Autodesk Fusion 360 part; units mm, degrees
note: some values were not read from the file. Set by a fixed rule: which face or edge a step refers to.
(part 5 of 12)
sketch "Sketch1" plane through (0, 0, 0) normal (0, 0, 1) x (1, 0, 0) in component "Component"
  spline S0 degree 5 poles (6.0486, -1.3928) (6.0487, -1.3928) (6.049, -1.3929) (6.0495, -1.393) (6.0503, -1.3931) (6.0514, -1.3934) (6.0527, -1.3936) (6.0541, -1.3939) (6.0558, -1.3942) (6.0576, -1.3945) (6.0596, -1.3948) (6.0618, -1.3952) (6.0641, -1.3955) (6.0665, -1.3959) (6.0692, -1.3963) (6.072, -1.3967) (6.0749, -1.3971) (6.078, -1.3975) (6.0812, -1.3979) (6.0846, -1.3983) (6.0881, -1.3987) (6.0918, -1.3991) (6.0956, -1.3995) (6.0995, -1.3999) (6.1036, -1.4002) (6.1078, -1.4006) (6.1121, -1.401) (6.1166, -1.4013) (6.1212, -1.4017) (6.1259, -1.402) (6.1308, -1.4023) (6.1357, -1.4026) (6.1408, -1.4029) (6.1461, -1.4032) (6.1514, -1.4034) (6.1569, -1.4036) (6.1624, -1.4038) (6.1681, -1.404) (6.1739, -1.4041) (6.1798, -1.4043) (6.1858, -1.4044) (6.192, -1.4044) (6.1982, -1.4045) (6.2046, -1.4045) (6.211, -1.4045) (6.2176, -1.4045) (6.2242, -1.4044) (6.231, -1.4043) (6.2379, -1.4042) (6.2448, -1.404) (6.2519, -1.4038) (6.259, -1.4036) (6.2663, -1.4033) (6.2736, -1.403) (6.2811, -1.4026) (6.2886, -1.4022) (6.2962, -1.4018) (6.304, -1.4014) (6.3118, -1.4009) (6.3197, -1.4003) (6.3277, -1.3997) (6.3357, -1.3991) (6.3439, -1.3985) (6.3522, -1.3978) (6.3605, -1.397) (6.3689, -1.3962) (6.3774, -1.3954) (6.386, -1.3945) (6.3946, -1.3936) (6.4034, -1.3926) (6.4122, -1.3916) (6.4211, -1.3905) (6.43, -1.3894) (6.4391, -1.3882) (6.4482, -1.387) (6.4574, -1.3858) (6.4667, -1.3845) (6.476, -1.3831) (6.4855, -1.3817) (6.4949, -1.3803) (6.5045, -1.3788) (6.5141, -1.3772) (6.5238, -1.3756) (6.5336, -1.3739) (6.5434, -1.3722) (6.5533, -1.3704) (6.5633, -1.3686) (6.5733, -1.3668) (6.5834, -1.3648) (6.5936, -1.3628) (6.6038, -1.3608) (6.6141, -1.3587) (6.6244, -1.3566) (6.6348, -1.3544) (6.6453, -1.3521) (6.6558, -1.3498) (6.6664, -1.3474) (6.6771, -1.345) (6.6878, -1.3425) (6.6985, -1.34) (6.7093, -1.3374) (6.7202, -1.3347) (6.7311, -1.332) (6.7421, -1.3292) (6.7531, -1.3264) (6.7642, -1.3235) (6.7754, -1.3206) (6.7865, -1.3176) (6.7978, -1.3145) (6.8091, -1.3114) (6.8204, -1.3082) (6.8318, -1.3049) (6.8432, -1.3016) (6.8547, -1.2982) (6.8663, -1.2948) (6.8778, -1.2913) (6.8895, -1.2878) (6.9011, -1.2842) (6.9129, -1.2805) (6.9246, -1.2767) (6.9364, -1.2729) (6.9483, -1.2691) (6.9602, -1.2651) (6.9721, -1.2611) (6.9841, -1.2571) (6.9961, -1.253) (7.0081, -1.2488) (7.0202, -1.2445) (7.0324, -1.2402) (7.0445, -1.2359) (7.0568, -1.2314) (7.069, -1.2269) (7.0813, -1.2224) (7.0936, -1.2177) (7.106, -1.213) (7.1184, -1.2083) (7.1308, -1.2035) (7.1433, -1.1986) (7.1558, -1.1936) (7.1683, -1.1886) (7.1809, -1.1835) (7.1935, -1.1784) (7.2061, -1.1731) (7.2188, -1.1679) (7.2314, -1.1625) (7.2442, -1.1571) (7.2569, -1.1516) (7.2697, -1.1461) (7.2825, -1.1405) (7.2953, -1.1348) (7.3082, -1.129) (7.3211, -1.1232) (7.334, -1.1173) (7.347, -1.1114) (7.36, -1.1054) (7.373, -1.0993) (7.386, -1.0932) (7.399, -1.0869) (7.4121, -1.0807) (7.4252, -1.0743) (7.4383, -1.0679) (7.4515, -1.0614) (7.4646, -1.0549) (7.4778, -1.0482) (7.491, -1.0416) (7.5043, -1.0348) (7.5175, -1.028) (7.5308, -1.0211) (7.5441, -1.0141) (7.5574, -1.0071) (7.5707, -1) (7.5841, -0.9929) (7.5974, -0.9856) (7.6108, -0.9783) (7.6242, -0.971) (7.6376, -0.9635) (7.6511, -0.956) (7.6645, -0.9484) (7.678, -0.9408) (7.6914, -0.9331) (7.7049, -0.9253) (7.7184, -0.9175) (7.732, -0.9096) (7.7455, -0.9016) (7.759, -0.8935) (7.7726, -0.8854) (7.7862, -0.8772) (7.7998, -0.869) (7.8134, -0.8606) (7.827, -0.8523) (7.8406, -0.8438) (7.8542, -0.8353) (7.8678, -0.8267) (7.8815, -0.818) (7.8951, -0.8093) (7.9088, -0.8004) (7.9225, -0.7916) (7.9361, -0.7826) (7.9498, -0.7736) (7.9635, -0.7645) (7.9772, -0.7554) (7.9909, -0.7462) (8.0046, -0.7369) (8.0183, -0.7275) (8.0321, -0.7181) (8.0458, -0.7086) (8.0595, -0.6991) (8.0732, -0.6894) (8.087, -0.6797) (8.1007, -0.67) (8.1145, -0.6601) (8.1282, -0.6502) (8.1419, -0.6402) (8.1557, -0.6302) (8.1694, -0.6201) (8.1832, -0.6099) (8.1969, -0.5997) (8.2107, -0.5894) (8.2244, -0.579) (8.2382, -0.5685) (8.2519, -0.558) (8.2657, -0.5474) (8.2794, -0.5368) (8.2932, -0.526) (8.3069, -0.5152) (8.3207, -0.5044) (8.3344, -0.4934) (8.3481, -0.4824) (8.3619, -0.4714) (8.3756, -0.4603) (8.3893, -0.449) (8.403, -0.4378) (8.4167, -0.4264) (8.4304, -0.415) (8.4441, -0.4036) (8.4578, -0.392) (8.4715, -0.3804) (8.4852, -0.3687) (8.4989, -0.357) (8.5125, -0.3452) (8.5262, -0.3333) (8.5371, -0.3238) (8.5453, -0.3166) (8.5507, -0.3117) (8.5535, -0.3093) knots 0 0 0 0 0 0 0.00416667 0.00833333 0.0125 0.01666667 0.02083333 0.025 0.02916667 0.03333333 0.0375 0.04166667 0.04583333 0.05 0.05416667 0.05833333 0.0625 0.06666667 0.07083333 0.075 0.07916667 0.08333333 0.0875 0.09166667 0.09583333 0.1 0.10416667 0.10833333 0.1125 0.11666667 0.12083333 0.125 0.12916667 0.13333333 0.1375 0.14166667 0.14583333 0.15 0.15416667 0.15833333 0.1625 0.16666667 0.17083333 0.175 0.17916667 0.18333333 0.1875 0.19166667 0.19583333 0.2 0.20416667 0.20833333 0.2125 0.21666667 0.22083333 0.225 0.22916667 0.23333333 0.2375 0.24166667 0.24583333 0.25 0.25416667 0.25833333 0.2625 0.26666667 0.27083333 0.275 0.27916667 0.28333333 0.2875 0.29166667 0.29583333 0.3 0.30416667 0.30833333 0.3125 0.31666667 0.32083333 0.325 0.32916667 0.33333333 0.3375 0.34166667 0.34583333 0.35 0.35416667 0.35833333 0.3625 0.36666667 0.37083333 0.375 0.37916667 0.38333333 0.3875 0.39166667 0.39583333 0.4 0.40416667 0.40833333 0.4125 0.41666667 0.42083333 0.425 0.42916667 0.43333333 0.4375 0.44166667 0.44583333 0.45 0.45416667 0.45833333 0.4625 0.46666667 0.47083333 0.475 0.47916667 0.48333333 0.4875 0.49166667 0.49583333 0.5 0.50416667 0.50833333 0.5125 0.51666667 0.52083333 0.525 0.52916667 0.53333333 0.5375 0.54166667 0.54583333 0.55 0.55416667 0.55833333 0.5625 0.56666667 0.57083333 0.575 0.57916667 0.58333333 0.5875 0.59166667 0.59583333 0.6 0.60416667 0.60833333 0.6125 0.61666667 0.62083333 0.625 0.62916667 0.63333333 0.6375 0.64166667 0.64583333 0.65 0.65416667 0.65833333 0.6625 0.66666667 0.67083333 0.675 0.67916667 0.68333333 0.6875 0.69166667 0.69583333 0.7 0.70416667 0.70833333 0.7125 0.71666667 0.72083333 0.725 0.72916667 0.73333333 0.7375 0.74166667 0.74583333 0.75 0.75416667 0.75833333 0.7625 0.76666667 0.77083333 0.775 0.77916667 0.78333333 0.7875 0.79166667 0.79583333 0.8 0.80416667 0.80833333 0.8125 0.81666667 0.82083333 0.825 0.82916667 0.83333333 0.8375 0.84166667 0.84583333 0.85 0.85416667 0.85833333 0.8625 0.86666667 0.87083333 0.875 0.87916667 0.88333333 0.8875 0.89166667 0.89583333 0.9 0.90416667 0.90833333 0.9125 0.91666667 0.92083333 0.925 0.92916667 0.93333333 0.9375 0.94166667 0.94583333 0.95 0.95416667 0.95833333 0.9625 0.96666667 0.97083333 0.975 0.97916667 0.98333333 0.9875 0.99166667 0.99583333 1 1 1 1 1 1
  spline S1 degree 5 poles (6.0486, 1.3928) (6.0487, 1.3928) (6.049, 1.3929) (6.0495, 1.393) (6.0503, 1.3931) (6.0514, 1.3934) (6.0527, 1.3936) (6.0541, 1.3939) (6.0558, 1.3942) (6.0576, 1.3945) (6.0596, 1.3948) (6.0618, 1.3952) (6.0641, 1.3955) (6.0665, 1.3959) (6.0692, 1.3963) (6.072, 1.3967) (6.0749, 1.3971) (6.078, 1.3975) (6.0812, 1.3979) (6.0846, 1.3983) (6.0881, 1.3987) (6.0918, 1.3991) (6.0956, 1.3995) (6.0995, 1.3999) (6.1036, 1.4002) (6.1078, 1.4006) (6.1121, 1.401) (6.1166, 1.4013) (6.1212, 1.4017) (6.1259, 1.402) (6.1308, 1.4023) (6.1357, 1.4026) (6.1408, 1.4029) (6.1461, 1.4032) (6.1514, 1.4034) (6.1569, 1.4036) (6.1624, 1.4038) (6.1681, 1.404) (6.1739, 1.4041) (6.1798, 1.4043) (6.1858, 1.4044) (6.192, 1.4044) (6.1982, 1.4045) (6.2046, 1.4045) (6.211, 1.4045) (6.2176, 1.4045) (6.2242, 1.4044) (6.231, 1.4043) (6.2379, 1.4042) (6.2448, 1.404) (6.2519, 1.4038) (6.259, 1.4036) (6.2663, 1.4033) (6.2736, 1.403) (6.2811, 1.4026) (6.2886, 1.4022) (6.2962, 1.4018) (6.304, 1.4014) (6.3118, 1.4009) (6.3197, 1.4003) (6.3277, 1.3997) (6.3357, 1.3991) (6.3439, 1.3985) (6.3522, 1.3978) (6.3605, 1.397) (6.3689, 1.3962) (6.3774, 1.3954) (6.386, 1.3945) (6.3946, 1.3936) (6.4034, 1.3926) (6.4122, 1.3916) (6.4211, 1.3905) (6.43, 1.3894) (6.4391, 1.3882) (6.4482, 1.387) (6.4574, 1.3858) (6.4667, 1.3845) (6.476, 1.3831) (6.4855, 1.3817) (6.4949, 1.3803) (6.5045, 1.3788) (6.5141, 1.3772) (6.5238, 1.3756) (6.5336, 1.3739) (6.5434, 1.3722) (6.5533, 1.3704) (6.5633, 1.3686) (6.5733, 1.3668) (6.5834, 1.3648) (6.5936, 1.3628) (6.6038, 1.3608) (6.6141, 1.3587) (6.6244, 1.3566) (6.6348, 1.3544) (6.6453, 1.3521) (6.6558, 1.3498) (6.6664, 1.3474) (6.6771, 1.345) (6.6878, 1.3425) (6.6985, 1.34) (6.7093, 1.3374) (6.7202, 1.3347) (6.7311, 1.332) (6.7421, 1.3292) (6.7531, 1.3264) (6.7642, 1.3235) (6.7754, 1.3206) (6.7865, 1.3176) (6.7978, 1.3145) (6.8091, 1.3114) (6.8204, 1.3082) (6.8318, 1.3049) (6.8432, 1.3016) (6.8547, 1.2982) (6.8663, 1.2948) (6.8778, 1.2913) (6.8895, 1.2878) (6.9011, 1.2842) (6.9129, 1.2805) (6.9246, 1.2767) (6.9364, 1.2729) (6.9483, 1.2691) (6.9602, 1.2651) (6.9721, 1.2611) (6.9841, 1.2571) (6.9961, 1.253) (7.0081, 1.2488) (7.0202, 1.2445) (7.0324, 1.2402) (7.0445, 1.2359) (7.0568, 1.2314) (7.069, 1.2269) (7.0813, 1.2224) (7.0936, 1.2177) (7.106, 1.213) (7.1184, 1.2083) (7.1308, 1.2035) (7.1433, 1.1986) (7.1558, 1.1936) (7.1683, 1.1886) (7.1809, 1.1835) (7.1935, 1.1784) (7.2061, 1.1731) (7.2188, 1.1679) (7.2314, 1.1625) (7.2442, 1.1571) (7.2569, 1.1516) (7.2697, 1.1461) (7.2825, 1.1405) (7.2953, 1.1348) (7.3082, 1.129) (7.3211, 1.1232) (7.334, 1.1173) (7.347, 1.1114) (7.36, 1.1054) (7.373, 1.0993) (7.386, 1.0932) (7.399, 1.0869) (7.4121, 1.0807) (7.4252, 1.0743) (7.4383, 1.0679) (7.4515, 1.0614) (7.4646, 1.0549) (7.4778, 1.0482) (7.491, 1.0416) (7.5043, 1.0348) (7.5175, 1.028) (7.5308, 1.0211) (7.5441, 1.0141) (7.5574, 1.0071) (7.5707, 1) (7.5841, 0.9929) (7.5974, 0.9856) (7.6108, 0.9783) (7.6242, 0.971) (7.6376, 0.9635) (7.6511, 0.956) (7.6645, 0.9484) (7.678, 0.9408) (7.6914, 0.9331) (7.7049, 0.9253) (7.7184, 0.9175) (7.732, 0.9096) (7.7455, 0.9016) (7.759, 0.8935) (7.7726, 0.8854) (7.7862, 0.8772) (7.7998, 0.869) (7.8134, 0.8606) (7.827, 0.8523) (7.8406, 0.8438) (7.8542, 0.8353) (7.8678, 0.8267) (7.8815, 0.818) (7.8951, 0.8093) (7.9088, 0.8004) (7.9225, 0.7916) (7.9361, 0.7826) (7.9498, 0.7736) (7.9635, 0.7645) (7.9772, 0.7554) (7.9909, 0.7462) (8.0046, 0.7369) (8.0183, 0.7275) (8.0321, 0.7181) (8.0458, 0.7086) (8.0595, 0.6991) (8.0732, 0.6894) (8.087, 0.6797) (8.1007, 0.67) (8.1145, 0.6601) (8.1282, 0.6502) (8.1419, 0.6402) (8.1557, 0.6302) (8.1694, 0.6201) (8.1832, 0.6099) (8.1969, 0.5997) (8.2107, 0.5894) (8.2244, 0.579) (8.2382, 0.5685) (8.2519, 0.558) (8.2657, 0.5474) (8.2794, 0.5368) (8.2932, 0.526) (8.3069, 0.5152) (8.3207, 0.5044) (8.3344, 0.4934) (8.3481, 0.4824) (8.3619, 0.4714) (8.3756, 0.4603) (8.3893, 0.449) (8.403, 0.4378) (8.4167, 0.4264) (8.4304, 0.415) (8.4441, 0.4036) (8.4578, 0.392) (8.4715, 0.3804) (8.4852, 0.3687) (8.4989, 0.357) (8.5125, 0.3452) (8.5262, 0.3333) (8.5371, 0.3238) (8.5453, 0.3166) (8.5507, 0.3117) (8.5535, 0.3093) knots 0 0 0 0 0 0 0.00416667 0.00833333 0.0125 0.01666667 0.02083333 0.025 0.02916667 0.03333333 0.0375 0.04166667 0.04583333 0.05 0.05416667 0.05833333 0.0625 0.06666667 0.07083333 0.075 0.07916667 0.08333333 0.0875 0.09166667 0.09583333 0.1 0.10416667 0.10833333 0.1125 0.11666667 0.12083333 0.125 0.12916667 0.13333333 0.1375 0.14166667 0.14583333 0.15 0.15416667 0.15833333 0.1625 0.16666667 0.17083333 0.175 0.17916667 0.18333333 0.1875 0.19166667 0.19583333 0.2 0.20416667 0.20833333 0.2125 0.21666667 0.22083333 0.225 0.22916667 0.23333333 0.2375 0.24166667 0.24583333 0.25 0.25416667 0.25833333 0.2625 0.26666667 0.27083333 0.275 0.27916667 0.28333333 0.2875 0.29166667 0.29583333 0.3 0.30416667 0.30833333 0.3125 0.31666667 0.32083333 0.325 0.32916667 0.33333333 0.3375 0.34166667 0.34583333 0.35 0.35416667 0.35833333 0.3625 0.36666667 0.37083333 0.375 0.37916667 0.38333333 0.3875 0.39166667 0.39583333 0.4 0.40416667 0.40833333 0.4125 0.41666667 0.42083333 0.425 0.42916667 0.43333333 0.4375 0.44166667 0.44583333 0.45 0.45416667 0.45833333 0.4625 0.46666667 0.47083333 0.475 0.47916667 0.48333333 0.4875 0.49166667 0.49583333 0.5 0.50416667 0.50833333 0.5125 0.51666667 0.52083333 0.525 0.52916667 0.53333333 0.5375 0.54166667 0.54583333 0.55 0.55416667 0.55833333 0.5625 0.56666667 0.57083333 0.575 0.57916667 0.58333333 0.5875 0.59166667 0.59583333 0.6 0.60416667 0.60833333 0.6125 0.61666667 0.62083333 0.625 0.62916667 0.63333333 0.6375 0.64166667 0.64583333 0.65 0.65416667 0.65833333 0.6625 0.66666667 0.67083333 0.675 0.67916667 0.68333333 0.6875 0.69166667 0.69583333 0.7 0.70416667 0.70833333 0.7125 0.71666667 0.72083333 0.725 0.72916667 0.73333333 0.7375 0.74166667 0.74583333 0.75 0.75416667 0.75833333 0.7625 0.76666667 0.77083333 0.775 0.77916667 0.78333333 0.7875 0.79166667 0.79583333 0.8 0.80416667 0.80833333 0.8125 0.81666667 0.82083333 0.825 0.82916667 0.83333333 0.8375 0.84166667 0.84583333 0.85 0.85416667 0.85833333 0.8625 0.86666667 0.87083333 0.875 0.87916667 0.88333333 0.8875 0.89166667 0.89583333 0.9 0.90416667 0.90833333 0.9125 0.91666667 0.92083333 0.925 0.92916667 0.93333333 0.9375 0.94166667 0.94583333 0.95 0.95416667 0.95833333 0.9625 0.96666667 0.97083333 0.975 0.97916667 0.98333333 0.9875 0.99166667 0.99583333 1 1 1 1 1 1
  spline S2 degree 5 poles (6.0475, -1.3925) (6.0475, -1.3926) (6.0476, -1.3926) (6.0477, -1.3926) (6.0479, -1.3926) (6.0481, -1.3927) (6.0483, -1.3927) (6.0485, -1.3928) (6.0485, -1.3928) (6.0486, -1.3928) knots 0 0 0 0 0 0 0.2 0.4 0.6 0.8 1 1 1 1 1 1
  spline S3 degree 5 poles (6.0475, 1.3925) (6.0475, 1.3926) (6.0476, 1.3926) (6.0477, 1.3926) (6.0479, 1.3926) (6.0481, 1.3927) (6.0483, 1.3927) (6.0485, 1.3928) (6.0485, 1.3928) (6.0486, 1.3928) knots 0 0 0 0 0 0 0.2 0.4 0.6 0.8 1 1 1 1 1 1
  line L0 (0, 0) -> (6.0475, -1.3925)
  line L1 (0, 0) -> (6.0475, 1.3925)
  arc A0 (8.5535, -0.3093) -> (8.5535, 0.3093) centre (0, 0) ccw
  point P0 (6.052, -1.3935)
  point P1 (6.0578, -1.3945)
  point P2 (6.0658, -1.3958)
  point P3 (6.0762, -1.3972)
  point P4 (6.089, -1.3988)
  point P5 (6.104, -1.4003)
  point P6 (6.1215, -1.4017)
  point P7 (6.1413, -1.4029)
  point P8 (6.1634, -1.4038)
  point P9 (6.1879, -1.4044)
  point P10 (6.2147, -1.4045)
  point P11 (6.2438, -1.404)
  point P12 (6.2753, -1.4029)
  point P13 (6.3091, -1.401)
  point P14 (6.3451, -1.3984)
  point P15 (6.3834, -1.3948)
  point P16 (6.424, -1.3902)
  point P17 (6.4667, -1.3845)
  point P18 (6.5117, -1.3776)
  point P19 (6.5588, -1.3694)
  point P20 (6.608, -1.36)
  point P21 (6.6593, -1.349)
  point P22 (6.7127, -1.3366)
  point P23 (6.7681, -1.3225)
  point P24 (6.8254, -1.3068)
  point P25 (6.8847, -1.2892)
  point P26 (6.9458, -1.2699)
  point P27 (7.0088, -1.2486)
  point P28 (7.0735, -1.2253)
  point P29 (7.1399, -1.1999)
  point P30 (7.208, -1.1723)
  point P31 (7.2777, -1.1426)
  point P32 (7.349, -1.1105)
  point P33 (7.4217, -1.076)
  point P34 (7.4958, -1.0391)
  point P35 (7.5712, -0.9997)
  point P36 (7.6479, -0.9578)
  point P37 (7.7258, -0.9131)
  point P38 (7.8049, -0.8658)
  point P39 (7.885, -0.8158)
  point P40 (7.966, -0.7629)
  point P41 (8.0479, -0.7071)
  point P42 (8.1307, -0.6484)
  point P43 (8.2141, -0.5867)
  point P44 (8.2982, -0.5221)
  point P45 (8.3829, -0.4543)
  point P46 (8.468, -0.3834)
  point P47 (6.052, 1.3935)
  point P48 (6.0578, 1.3945)
  point P49 (6.0658, 1.3958)
  point P50 (6.0762, 1.3972)
  point P51 (6.089, 1.3988)
  point P52 (6.104, 1.4003)
  point P53 (6.1215, 1.4017)
  point P54 (6.1413, 1.4029)
  point P55 (6.1634, 1.4038)
  point P56 (6.1879, 1.4044)
  point P57 (6.2147, 1.4045)
  point P58 (6.2438, 1.404)
  point P59 (6.2753, 1.4029)
  point P60 (6.3091, 1.401)
  point P61 (6.3451, 1.3984)
  point P62 (6.3834, 1.3948)
  point P63 (6.424, 1.3902)
  point P64 (6.4667, 1.3845)
  point P65 (6.5117, 1.3776)
  point P66 (6.5588, 1.3694)
  point P67 (6.608, 1.36)
  point P68 (6.6593, 1.349)
  point P69 (6.7127, 1.3366)
  point P70 (6.7681, 1.3225)
  point P71 (6.8254, 1.3068)
  point P72 (6.8847, 1.2892)
  point P73 (6.9458, 1.2699)
  point P74 (7.0088, 1.2486)
  point P75 (7.0735, 1.2253)
  point P76 (7.1399, 1.1999)
  point P77 (7.208, 1.1723)
  point P78 (7.2777, 1.1426)
  point P79 (7.349, 1.1105)
  point P80 (7.4217, 1.076)
  point P81 (7.4958, 1.0391)
  point P82 (7.5712, 0.9997)
  point P83 (7.6479, 0.9578)
  point P84 (7.7258, 0.9131)
  point P85 (7.8049, 0.8658)
  point P86 (7.885, 0.8158)
  point P87 (7.966, 0.7629)
  point P88 (8.0479, 0.7071)
  point P89 (8.1307, 0.6484)
  point P90 (8.2141, 0.5867)
  point P91 (8.2982, 0.5221)
  point P92 (8.3829, 0.4543)
  point P93 (8.468, 0.3834)
sketch "Sketch2" plane through (0, 0, 0) normal (0, 0, 1) x (1, 0, 0) in component "Component"
  circle A0 centre (0, 0) radius 4.7075
extrude "Extrude1" add sketch "Sketch2" along normal blind 3 makes body 1 in component "Component"
extrude "Extrude2" add sketch "Sketch1" along normal blind 3 separate body makes body 2 in component "Component"
pattern_circular "C-Pattern1" count 8 over 360 about axis through (0, 0, 1.75) along (0, 0, 1) of "Extrude2" makes body 3 at (1.754, 1.0974, 1) makes body 4 at (0.4643, 2.0162, 1) makes body 5 at (-1.0974, 1.754, 1) makes body 6 at (-2.0162, 0.4643, 1) makes body 7 at (-1.754, -1.0974, 1) makes body 8 at (0.4643, -2.0162, 1) makes body 9 at (1.0974, -1.754, 1) in component "Component"
combine "Combine1" operation add target body 1 tool bodies 2 3 4 5 6 7 8 9 in component "Component"
sketch "Sketch3" plane through (0, 0, 0) normal (0, 0, 1) x (1, 0, 0) in component "Component"
  line L0 (0, 0) -> (50.8154, 0) construction
  line L1 (50.8154, 0) -> (50.8154, 3) construction
  line L2 (50.8154, 3) -> (0, 3) construction
  line L3 (0, 3) -> (0, 0) construction
  constraint perpendicular L0 L1
  constraint parallel L0 L2
  constraint parallel L1 L3
sketch "Sketch3 (2)" plane through (0, 0, 3) normal (0, 0, 1) x (-1, 0, 0)
  arc A0 (-3.9908, 2.4969) -> (-4.5874, 1.0563) centre (0, 0) ccw
  line L0 (-4.5874, 1.0563) -> (-6.0475, 1.3925)
  line L1 (-6.0475, 1.3925) -> (-6.0486, 1.3928)
  spline S0 degree 5 poles (-6.0486, 1.3928) (-6.0487, 1.3928) (-6.049, 1.3929) (-6.0495, 1.393) (-6.0503, 1.3931) (-6.0514, 1.3934) (-6.0527, 1.3936) (-6.0541, 1.3939) (-6.0558, 1.3942) (-6.0576, 1.3945) (-6.0596, 1.3948) (-6.0618, 1.3952) (-6.0641, 1.3955) (-6.0665, 1.3959) (-6.0692, 1.3963) (-6.072, 1.3967) (-6.0749, 1.3971) (-6.078, 1.3975) (-6.0812, 1.3979) (-6.0846, 1.3983) (-6.0881, 1.3987) (-6.0918, 1.3991) (-6.0956, 1.3995) (-6.0995, 1.3999) (-6.1036, 1.4002) (-6.1078, 1.4006) (-6.1121, 1.401) (-6.1166, 1.4013) (-6.1212, 1.4017) (-6.1259, 1.402) (-6.1308, 1.4023) (-6.1357, 1.4026) (-6.1408, 1.4029) (-6.1461, 1.4032) (-6.1514, 1.4034) (-6.1569, 1.4036) (-6.1624, 1.4038) (-6.1681, 1.404) (-6.1739, 1.4041) (-6.1798, 1.4043) (-6.1858, 1.4044) (-6.192, 1.4044) (-6.1982, 1.4045) (-6.2046, 1.4045) (-6.211, 1.4045) (-6.2176, 1.4045) (-6.2242, 1.4044) (-6.231, 1.4043) (-6.2379, 1.4042) (-6.2448, 1.404) (-6.2519, 1.4038) (-6.259, 1.4036) (-6.2663, 1.4033) (-6.2736, 1.403) (-6.2811, 1.4026) (-6.2886, 1.4022) (-6.2962, 1.4018) (-6.304, 1.4014) (-6.3118, 1.4009) (-6.3197, 1.4003) (-6.3277, 1.3997) (-6.3357, 1.3991) (-6.3439, 1.3985) (-6.3522, 1.3978) (-6.3605, 1.397) (-6.3689, 1.3962) (-6.3774, 1.3954) (-6.386, 1.3945) (-6.3946, 1.3936) (-6.4034, 1.3926) (-6.4122, 1.3916) (-6.4211, 1.3905) (-6.43, 1.3894) (-6.4391, 1.3882) (-6.4482, 1.387) (-6.4574, 1.3858) (-6.4667, 1.3845) (-6.476, 1.3831) (-6.4855, 1.3817) (-6.4949, 1.3803) (-6.5045, 1.3788) (-6.5141, 1.3772) (-6.5238, 1.3756) (-6.5336, 1.3739) (-6.5434, 1.3722) (-6.5533, 1.3704) (-6.5633, 1.3686) (-6.5733, 1.3668) (-6.5834, 1.3648) (-6.5936, 1.3628) (-6.6038, 1.3608) (-6.6141, 1.3587) (-6.6244, 1.3566) (-6.6348, 1.3544) (-6.6453, 1.3521) (-6.6558, 1.3498) (-6.6664, 1.3474) (-6.6771, 1.345) (-6.6878, 1.3425) (-6.6985, 1.34) (-6.7093, 1.3374) (-6.7202, 1.3347) (-6.7311, 1.332) (-6.7421, 1.3292) (-6.7531, 1.3264) (-6.7642, 1.3235) (-6.7754, 1.3206) (-6.7865, 1.3176) (-6.7978, 1.3145) (-6.8091, 1.3114) (-6.8204, 1.3082) (-6.8318, 1.3049) (-6.8432, 1.3016) (-6.8547, 1.2982) (-6.8663, 1.2948) (-6.8778, 1.2913) (-6.8895, 1.2878) (-6.9011, 1.2842) (-6.9129, 1.2805) (-6.9246, 1.2767) (-6.9364, 1.2729) (-6.9483, 1.2691) (-6.9602, 1.2651) (-6.9721, 1.2611) (-6.9841, 1.2571) (-6.9961, 1.253) (-7.0081, 1.2488) (-7.0202, 1.2445) (-7.0324, 1.2402) (-7.0445, 1.2359) (-7.0568, 1.2314) (-7.069, 1.2269) (-7.0813, 1.2224) (-7.0936, 1.2177) (-7.106, 1.213) (-7.1184, 1.2083) (-7.1308, 1.2035) (-7.1433, 1.1986) (-7.1558, 1.1936) (-7.1683, 1.1886) (-7.1809, 1.1835) (-7.1935, 1.1784) (-7.2061, 1.1731) (-7.2188, 1.1679) (-7.2314, 1.1625) (-7.2442, 1.1571) (-7.2569, 1.1516) (-7.2697, 1.1461) (-7.2825, 1.1405) (-7.2953, 1.1348) (-7.3082, 1.129) (-7.3211, 1.1232) (-7.334, 1.1173) (-7.347, 1.1114) (-7.36, 1.1054) (-7.373, 1.0993) (-7.386, 1.0932) (-7.399, 1.0869) (-7.4121, 1.0807) (-7.4252, 1.0743) (-7.4383, 1.0679) (-7.4515, 1.0614) (-7.4646, 1.0549) (-7.4778, 1.0482) (-7.491, 1.0416) (-7.5043, 1.0348) (-7.5175, 1.028) (-7.5308, 1.0211) (-7.5441, 1.0141) (-7.5574, 1.0071) (-7.5707, 1) (-7.5841, 0.9929) (-7.5974, 0.9856) (-7.6108, 0.9783) (-7.6242, 0.971) (-7.6376, 0.9635) (-7.6511, 0.956) (-7.6645, 0.9484) (-7.678, 0.9408) (-7.6914, 0.9331) (-7.7049, 0.9253) (-7.7184, 0.9175) (-7.732, 0.9096) (-7.7455, 0.9016) (-7.759, 0.8935) (-7.7726, 0.8854) (-7.7862, 0.8772) (-7.7998, 0.869) (-7.8134, 0.8606) (-7.827, 0.8523) (-7.8406, 0.8438) (-7.8542, 0.8353) (-7.8678, 0.8267) (-7.8815, 0.818) (-7.8951, 0.8093) (-7.9088, 0.8004) (-7.9225, 0.7916) (-7.9361, 0.7826) (-7.9498, 0.7736) (-7.9635, 0.7645) (-7.9772, 0.7554) (-7.9909, 0.7462) (-8.0046, 0.7369) (-8.0183, 0.7275) (-8.0321, 0.7181) (-8.0458, 0.7086) (-8.0595, 0.6991) (-8.0732, 0.6894) (-8.087, 0.6797) (-8.1007, 0.67) (-8.1145, 0.6601) (-8.1282, 0.6502) (-8.1419, 0.6402) (-8.1557, 0.6302) (-8.1694, 0.6201) (-8.1832, 0.6099) (-8.1969, 0.5997) (-8.2107, 0.5894) (-8.2244, 0.579) (-8.2382, 0.5685) (-8.2519, 0.558) (-8.2657, 0.5474) (-8.2794, 0.5368) (-8.2932, 0.526) (-8.3069, 0.5152) (-8.3207, 0.5044) (-8.3344, 0.4934) (-8.3481, 0.4824) (-8.3619, 0.4714) (-8.3756, 0.4603) (-8.3893, 0.449) (-8.403, 0.4378) (-8.4167, 0.4264) (-8.4304, 0.415) (-8.4441, 0.4036) (-8.4578, 0.392) (-8.4715, 0.3804) (-8.4852, 0.3687) (-8.4989, 0.357) (-8.5125, 0.3452) (-8.5262, 0.3333) (-8.5371, 0.3238) (-8.5453, 0.3166) (-8.5507, 0.3117) (-8.5535, 0.3093) knots 0 0 0 0 0 0 0.00416667 0.00833333 0.0125 0.01666667 0.02083333 0.025 0.02916667 0.03333333 0.0375 0.04166667 0.04583333 0.05 0.05416667 0.05833333 0.0625 0.06666667 0.07083333 0.075 0.07916667 0.08333333 0.0875 0.09166667 0.09583333 0.1 0.10416667 0.10833333 0.1125 0.11666667 0.12083333 0.125 0.12916667 0.13333333 0.1375 0.14166667 0.14583333 0.15 0.15416667 0.15833333 0.1625 0.16666667 0.17083333 0.175 0.17916667 0.18333333 0.1875 0.19166667 0.19583333 0.2 0.20416667 0.20833333 0.2125 0.21666667 0.22083333 0.225 0.22916667 0.23333333 0.2375 0.24166667 0.24583333 0.25 0.25416667 0.25833333 0.2625 0.26666667 0.27083333 0.275 0.27916667 0.28333333 0.2875 0.29166667 0.29583333 0.3 0.30416667 0.30833333 0.3125 0.31666667 0.32083333 0.325 0.32916667 0.33333333 0.3375 0.34166667 0.34583333 0.35 0.35416667 0.35833333 0.3625 0.36666667 0.37083333 0.375 0.37916667 0.38333333 0.3875 0.39166667 0.39583333 0.4 0.40416667 0.40833333 0.4125 0.41666667 0.42083333 0.425 0.42916667 0.43333333 0.4375 0.44166667 0.44583333 0.45 0.45416667 0.45833333 0.4625 0.46666667 0.47083333 0.475 0.47916667 0.48333333 0.4875 0.49166667 0.49583333 0.5 0.50416667 0.50833333 0.5125 0.51666667 0.52083333 0.525 0.52916667 0.53333333 0.5375 0.54166667 0.54583333 0.55 0.55416667 0.55833333 0.5625 0.56666667 0.57083333 0.575 0.57916667 0.58333333 0.5875 0.59166667 0.59583333 0.6 0.60416667 0.60833333 0.6125 0.61666667 0.62083333 0.625 0.62916667 0.63333333 0.6375 0.64166667 0.64583333 0.65 0.65416667 0.65833333 0.6625 0.66666667 0.67083333 0.675 0.67916667 0.68333333 0.6875 0.69166667 0.69583333 0.7 0.70416667 0.70833333 0.7125 0.71666667 0.72083333 0.725 0.72916667 0.73333333 0.7375 0.74166667 0.74583333 0.75 0.75416667 0.75833333 0.7625 0.76666667 0.77083333 0.775 0.77916667 0.78333333 0.7875 0.79166667 0.79583333 0.8 0.80416667 0.80833333 0.8125 0.81666667 0.82083333 0.825 0.82916667 0.83333333 0.8375 0.84166667 0.84583333 0.85 0.85416667 0.85833333 0.8625 0.86666667 0.87083333 0.875 0.87916667 0.88333333 0.8875 0.89166667 0.89583333 0.9 0.90416667 0.90833333 0.9125 0.91666667 0.92083333 0.925 0.92916667 0.93333333 0.9375 0.94166667 0.94583333 0.95 0.95416667 0.95833333 0.9625 0.96666667 0.97083333 0.975 0.97916667 0.98333333 0.9875 0.99166667 0.99583333 1 1 1 1 1 1
  arc A1 (-8.5535, 0.3093) -> (-8.5535, -0.3093) centre (0, 0) ccw
  spline S1 degree 5 poles (-8.5535, -0.3093) (-8.5507, -0.3117) (-8.5453, -0.3166) (-8.5371, -0.3238) (-8.5262, -0.3333) (-8.5125, -0.3452) (-8.4989, -0.357) (-8.4852, -0.3687) (-8.4715, -0.3804) (-8.4578, -0.392) (-8.4441, -0.4036) (-8.4304, -0.415) (-8.4167, -0.4264) (-8.403, -0.4378) (-8.3893, -0.449) (-8.3756, -0.4603) (-8.3619, -0.4714) (-8.3481, -0.4824) (-8.3344, -0.4934) (-8.3207, -0.5044) (-8.3069, -0.5152) (-8.2932, -0.526) (-8.2794, -0.5368) (-8.2657, -0.5474) (-8.2519, -0.558) (-8.2382, -0.5685) (-8.2244, -0.579) (-8.2107, -0.5894) (-8.1969, -0.5997) (-8.1832, -0.6099) (-8.1694, -0.6201) (-8.1557, -0.6302) (-8.1419, -0.6402) (-8.1282, -0.6502) (-8.1145, -0.6601) (-8.1007, -0.67) (-8.087, -0.6797) (-8.0732, -0.6894) (-8.0595, -0.6991) (-8.0458, -0.7086) (-8.0321, -0.7181) (-8.0183, -0.7275) (-8.0046, -0.7369) (-7.9909, -0.7462) (-7.9772, -0.7554) (-7.9635, -0.7645) (-7.9498, -0.7736) (-7.9361, -0.7826) (-7.9225, -0.7916) (-7.9088, -0.8004) (-7.8951, -0.8093) (-7.8815, -0.818) (-7.8678, -0.8267) (-7.8542, -0.8353) (-7.8406, -0.8438) (-7.827, -0.8523) (-7.8134, -0.8606) (-7.7998, -0.869) (-7.7862, -0.8772) (-7.7726, -0.8854) (-7.759, -0.8935) (-7.7455, -0.9016) (-7.732, -0.9096) (-7.7184, -0.9175) (-7.7049, -0.9253) (-7.6914, -0.9331) (-7.678, -0.9408) (-7.6645, -0.9484) (-7.6511, -0.956) (-7.6376, -0.9635) (-7.6242, -0.971) (-7.6108, -0.9783) (-7.5974, -0.9856) (-7.5841, -0.9929) (-7.5707, -1) (-7.5574, -1.0071) (-7.5441, -1.0141) (-7.5308, -1.0211) (-7.5175, -1.028) (-7.5043, -1.0348) (-7.491, -1.0416) (-7.4778, -1.0482) (-7.4646, -1.0549) (-7.4515, -1.0614) (-7.4383, -1.0679) (-7.4252, -1.0743) (-7.4121, -1.0807) (-7.399, -1.0869) (-7.386, -1.0932) (-7.373, -1.0993) (-7.36, -1.1054) (-7.347, -1.1114) (-7.334, -1.1173) (-7.3211, -1.1232) (-7.3082, -1.129) (-7.2953, -1.1348) (-7.2825, -1.1405) (-7.2697, -1.1461) (-7.2569, -1.1516) (-7.2442, -1.1571) (-7.2314, -1.1625) (-7.2188, -1.1679) (-7.2061, -1.1731) (-7.1935, -1.1784) (-7.1809, -1.1835) (-7.1683, -1.1886) (-7.1558, -1.1936) (-7.1433, -1.1986) (-7.1308, -1.2035) (-7.1184, -1.2083) (-7.106, -1.213) (-7.0936, -1.2177) (-7.0813, -1.2224) (-7.069, -1.2269) (-7.0568, -1.2314) (-7.0445, -1.2359) (-7.0324, -1.2402) (-7.0202, -1.2445) (-7.0081, -1.2488) (-6.9961, -1.253) (-6.9841, -1.2571) (-6.9721, -1.2611) (-6.9602, -1.2651) (-6.9483, -1.2691) (-6.9364, -1.2729) (-6.9246, -1.2767) (-6.9129, -1.2805) (-6.9011, -1.2842) (-6.8895, -1.2878) (-6.8778, -1.2913) (-6.8663, -1.2948) (-6.8547, -1.2982) (-6.8432, -1.3016) (-6.8318, -1.3049) (-6.8204, -1.3082) (-6.8091, -1.3114) (-6.7978, -1.3145) (-6.7865, -1.3176) (-6.7754, -1.3206) (-6.7642, -1.3235) (-6.7531, -1.3264) (-6.7421, -1.3292) (-6.7311, -1.332) (-6.7202, -1.3347) (-6.7093, -1.3374) (-6.6985, -1.34) (-6.6878, -1.3425) (-6.6771, -1.345) (-6.6664, -1.3474) (-6.6558, -1.3498) (-6.6453, -1.3521) (-6.6348, -1.3544) (-6.6244, -1.3566) (-6.6141, -1.3587) (-6.6038, -1.3608) (-6.5936, -1.3628) (-6.5834, -1.3648) (-6.5733, -1.3668) (-6.5633, -1.3686) (-6.5533, -1.3704) (-6.5434, -1.3722) (-6.5336, -1.3739) (-6.5238, -1.3756) (-6.5141, -1.3772) (-6.5045, -1.3788) (-6.4949, -1.3803) (-6.4855, -1.3817) (-6.476, -1.3831) (-6.4667, -1.3845) (-6.4574, -1.3858) (-6.4482, -1.387) (-6.4391, -1.3882) (-6.43, -1.3894) (-6.4211, -1.3905) (-6.4122, -1.3916) (-6.4034, -1.3926) (-6.3946, -1.3936) (-6.386, -1.3945) (-6.3774, -1.3954) (-6.3689, -1.3962) (-6.3605, -1.397) (-6.3522, -1.3978) (-6.3439, -1.3985) (-6.3357, -1.3991) (-6.3277, -1.3997) (-6.3197, -1.4003) (-6.3118, -1.4009) (-6.304, -1.4014) (-6.2962, -1.4018) (-6.2886, -1.4022) (-6.2811, -1.4026) (-6.2736, -1.403) (-6.2663, -1.4033) (-6.259, -1.4036) (-6.2519, -1.4038) (-6.2448, -1.404) (-6.2379, -1.4042) (-6.231, -1.4043) (-6.2242, -1.4044) (-6.2176, -1.4045) (-6.211, -1.4045) (-6.2046, -1.4045) (-6.1982, -1.4045) (-6.192, -1.4044) (-6.1858, -1.4044) (-6.1798, -1.4043) (-6.1739, -1.4041) (-6.1681, -1.404) (-6.1624, -1.4038) (-6.1569, -1.4036) (-6.1514, -1.4034) (-6.1461, -1.4032) (-6.1408, -1.4029) (-6.1357, -1.4026) (-6.1308, -1.4023) (-6.1259, -1.402) (-6.1212, -1.4017) (-6.1166, -1.4013) (-6.1121, -1.401) (-6.1078, -1.4006) (-6.1036, -1.4002) (-6.0995, -1.3999) (-6.0956, -1.3995) (-6.0918, -1.3991) (-6.0881, -1.3987) (-6.0846, -1.3983) (-6.0812, -1.3979) (-6.078, -1.3975) (-6.0749, -1.3971) (-6.072, -1.3967) (-6.0692, -1.3963) (-6.0665, -1.3959) (-6.0641, -1.3955) (-6.0618, -1.3952) (-6.0596, -1.3948) (-6.0576, -1.3945) (-6.0558, -1.3942) (-6.0541, -1.3939) (-6.0527, -1.3936) (-6.0514, -1.3934) (-6.0503, -1.3931) (-6.0495, -1.393) (-6.049, -1.3929) (-6.0487, -1.3928) (-6.0486, -1.3928) knots -1 -1 -1 -1 -1 -1 -0.99583333 -0.99166667 -0.9875 -0.98333333 -0.97916667 -0.975 -0.97083333 -0.96666667 -0.9625 -0.95833333 -0.95416667 -0.95 -0.94583333 -0.94166667 -0.9375 -0.93333333 -0.92916667 -0.925 -0.92083333 -0.91666667 -0.9125 -0.90833333 -0.90416667 -0.9 -0.89583333 -0.89166667 -0.8875 -0.88333333 -0.87916667 -0.875 -0.87083333 -0.86666667 -0.8625 -0.85833333 -0.85416667 -0.85 -0.84583333 -0.84166667 -0.8375 -0.83333333 -0.82916667 -0.825 -0.82083333 -0.81666667 -0.8125 -0.80833333 -0.80416667 -0.8 -0.79583333 -0.79166667 -0.7875 -0.78333333 -0.77916667 -0.775 -0.77083333 -0.76666667 -0.7625 -0.75833333 -0.75416667 -0.75 -0.74583333 -0.74166667 -0.7375 -0.73333333 -0.72916667 -0.725 -0.72083333 -0.71666667 -0.7125 -0.70833333 -0.70416667 -0.7 -0.69583333 -0.69166667 -0.6875 -0.68333333 -0.67916667 -0.675 -0.67083333 -0.66666667 -0.6625 -0.65833333 -0.65416667 -0.65 -0.64583333 -0.64166667 -0.6375 -0.63333333 -0.62916667 -0.625 -0.62083333 -0.61666667 -0.6125 -0.60833333 -0.60416667 -0.6 -0.59583333 -0.59166667 -0.5875 -0.58333333 -0.57916667 -0.575 -0.57083333 -0.56666667 -0.5625 -0.55833333 -0.55416667 -0.55 -0.54583333 -0.54166667 -0.5375 -0.53333333 -0.52916667 -0.525 -0.52083333 -0.51666667 -0.5125 -0.50833333 -0.50416667 -0.5 -0.49583333 -0.49166667 -0.4875 -0.48333333 -0.47916667 -0.475 -0.47083333 -0.46666667 -0.4625 -0.45833333 -0.45416667 -0.45 -0.44583333 -0.44166667 -0.4375 -0.43333333 -0.42916667 -0.425 -0.42083333 -0.41666667 -0.4125 -0.40833333 -0.40416667 -0.4 -0.39583333 -0.39166667 -0.3875 -0.38333333 -0.37916667 -0.375 -0.37083333 -0.36666667 -0.3625 -0.35833333 -0.35416667 -0.35 -0.34583333 -0.34166667 -0.3375 -0.33333333 -0.32916667 -0.325 -0.32083333 -0.31666667 -0.3125 -0.30833333 -0.30416667 -0.3 -0.29583333 -0.29166667 -0.2875 -0.28333333 -0.27916667 -0.275 -0.27083333 -0.26666667 -0.2625 -0.25833333 -0.25416667 -0.25 -0.24583333 -0.24166667 -0.2375 -0.23333333 -0.22916667 -0.225 -0.22083333 -0.21666667 -0.2125 -0.20833333 -0.20416667 -0.2 -0.19583333 -0.19166667 -0.1875 -0.18333333 -0.17916667 -0.175 -0.17083333 -0.16666667 -0.1625 -0.15833333 -0.15416667 -0.15 -0.14583333 -0.14166667 -0.1375 -0.13333333 -0.12916667 -0.125 -0.12083333 -0.11666667 -0.1125 -0.10833333 -0.10416667 -0.1 -0.09583333 -0.09166667 -0.0875 -0.08333333 -0.07916667 -0.075 -0.07083333 -0.06666667 -0.0625 -0.05833333 -0.05416667 -0.05 -0.04583333 -0.04166667 -0.0375 -0.03333333 -0.02916667 -0.025 -0.02083333 -0.01666667 -0.0125 -0.00833333 -0.00416667 0 0 0 0 0 0
  line L2 (-6.0486, -1.3928) -> (-6.0475, -1.3925)
  line L3 (-6.0475, -1.3925) -> (-4.5874, -1.0563)
  arc A2 (-4.5874, -1.0563) -> (-3.9908, -2.4969) centre (0, 0) ccw
  line L4 (-3.9908, -2.4969) -> (-5.2609, -3.2915)
  line L5 (-5.2609, -3.2915) -> (-5.2619, -3.2921)
  spline S2 degree 5 poles (-5.2619, -3.2921) (-5.262, -3.2922) (-5.2622, -3.2924) (-5.2626, -3.2927) (-5.2633, -3.2931) (-5.2642, -3.2937) (-5.2653, -3.2945) (-5.2665, -3.2953) (-5.2679, -3.2963) (-5.2694, -3.2973) (-5.2711, -3.2985) (-5.2728, -3.2998) (-5.2747, -3.3012) (-5.2767, -3.3026) (-5.2789, -3.3042) (-5.2811, -3.3059) (-5.2835, -3.3077) (-5.2859, -3.3096) (-5.2885, -3.3116) (-5.2912, -3.3137) (-5.294, -3.3159) (-5.2968, -3.3182) (-5.2998, -3.3206) (-5.3029, -3.3231) (-5.306, -3.3258) (-5.3092, -3.3285) (-5.3126, -3.3313) (-5.316, -3.3342) (-5.3195, -3.3372) (-5.323, -3.3403) (-5.3267, -3.3435) (-5.3304, -3.3468) (-5.3342, -3.3502) (-5.3381, -3.3537) (-5.342, -3.3573) (-5.3461, -3.361) (-5.3501, -3.3648) (-5.3543, -3.3687) (-5.3585, -3.3727) (-5.3628, -3.3768) (-5.3671, -3.381) (-5.3715, -3.3853) (-5.3759, -3.3897) (-5.3804, -3.3941) (-5.385, -3.3987) (-5.3896, -3.4034) (-5.3943, -3.4081) (-5.399, -3.413) (-5.4037, -3.4179) (-5.4085, -3.423) (-5.4134, -3.4281) (-5.4183, -3.4333) (-5.4232, -3.4387) (-5.4282, -3.4441) (-5.4332, -3.4496) (-5.4383, -3.4552) (-5.4434, -3.4609) (-5.4485, -3.4667) (-5.4537, -3.4725) (-5.4589, -3.4785) (-5.4641, -3.4846) (-5.4694, -3.4907) (-5.4747, -3.497) (-5.48, -3.5033) (-5.4854, -3.5097) (-5.4908, -3.5162) (-5.4962, -3.5228) (-5.5016, -3.5295) (-5.5071, -3.5363) (-5.5126, -3.5431) (-5.5181, -3.5501) (-5.5236, -3.5571) (-5.5292, -3.5643) (-5.5348, -3.5715) (-5.5404, -3.5788) (-5.546, -3.5862) (-5.5516, -3.5937) (-5.5573, -3.6012) (-5.5629, -3.6089) (-5.5686, -3.6166) (-5.5743, -3.6244) (-5.58, -3.6324) (-5.5857, -3.6404) (-5.5915, -3.6484) (-5.5972, -3.6566) (-5.603, -3.6648) (-5.6087, -3.6732) (-5.6145, -3.6816) (-5.6203, -3.6901) (-5.626, -3.6987) (-5.6318, -3.7073) (-5.6376, -3.7161) (-5.6434, -3.7249) (-5.6492, -3.7338) (-5.655, -3.7428) (-5.6608, -3.7519) (-5.6666, -3.7611) (-5.6725, -3.7703) (-5.6783, -3.7796) (-5.6841, -3.7891) (-5.6899, -3.7985) (-5.6957, -3.8081) (-5.7015, -3.8177) (-5.7073, -3.8275) (-5.7131, -3.8373) (-5.7189, -3.8472) (-5.7247, -3.8571) (-5.7305, -3.8672) (-5.7363, -3.8773) (-5.742, -3.8875) (-5.7478, -3.8977) (-5.7535, -3.9081) (-5.7593, -3.9185) (-5.765, -3.929) (-5.7708, -3.9396) (-5.7765, -3.9503) (-5.7822, -3.961) (-5.7879, -3.9718) (-5.7936, -3.9827) (-5.7992, -3.9937) (-5.8049, -4.0047) (-5.8105, -4.0158) (-5.8162, -4.027) (-5.8218, -4.0383) (-5.8274, -4.0496) (-5.833, -4.061) (-5.8385, -4.0725) (-5.8441, -4.084) (-5.8496, -4.0957) (-5.8551, -4.1074) (-5.8606, -4.1191) (-5.8661, -4.131) (-5.8716, -4.1429) (-5.877, -4.1549) (-5.8824, -4.1669) (-5.8878, -4.1791) (-5.8932, -4.1913) (-5.8986, -4.2035) (-5.9039, -4.2159) (-5.9092, -4.2283) (-5.9145, -4.2408) (-5.9198, -4.2533) (-5.925, -4.2659) (-5.9302, -4.2786) (-5.9354, -4.2914) (-5.9406, -4.3042) (-5.9457, -4.3171) (-5.9509, -4.3301) (-5.9559, -4.3431) (-5.961, -4.3562) (-5.966, -4.3693) (-5.971, -4.3826) (-5.976, -4.3959) (-5.981, -4.4092) (-5.9859, -4.4226) (-5.9908, -4.4361) (-5.9957, -4.4497) (-6.0005, -4.4633) (-6.0053, -4.477) (-6.0101, -4.4908) (-6.0148, -4.5046) (-6.0195, -4.5184) (-6.0242, -4.5324) (-6.0288, -4.5464) (-6.0335, -4.5605) (-6.038, -4.5746) (-6.0426, -4.5888) (-6.0471, -4.603) (-6.0516, -4.6174) (-6.056, -4.6317) (-6.0604, -4.6462) (-6.0648, -4.6607) (-6.0691, -4.6753) (-6.0734, -4.6899) (-6.0777, -4.7046) (-6.0819, -4.7193) (-6.0861, -4.7341) (-6.0903, -4.749) (-6.0944, -4.7639) (-6.0985, -4.7789) (-6.1025, -4.7939) (-6.1065, -4.809) (-6.1105, -4.8242) (-6.1144, -4.8394) (-6.1183, -4.8547) (-6.1221, -4.87) (-6.126, -4.8854) (-6.1297, -4.9008) (-6.1334, -4.9163) (-6.1371, -4.9319) (-6.1408, -4.9475) (-6.1444, -4.9631) (-6.1479, -4.9789) (-6.1515, -4.9946) (-6.1549, -5.0105) (-6.1584, -5.0264) (-6.1618, -5.0423) (-6.1651, -5.0583) (-6.1684, -5.0743) (-6.1717, -5.0904) (-6.1749, -5.1066) (-6.1781, -5.1228) (-6.1812, -5.1391) (-6.1843, -5.1554) (-6.1873, -5.1717) (-6.1903, -5.1882) (-6.1932, -5.2046) (-6.1961, -5.2211) (-6.199, -5.2377) (-6.2018, -5.2543) (-6.2046, -5.271) (-6.2073, -5.2877) (-6.2099, -5.3045) (-6.2126, -5.3213) (-6.2151, -5.3382) (-6.2177, -5.3551) (-6.2201, -5.3721) (-6.2226, -5.3891) (-6.225, -5.4062) (-6.2273, -5.4233) (-6.2296, -5.4404) (-6.2318, -5.4576) (-6.234, -5.4749) (-6.2361, -5.4922) (-6.2382, -5.5095) (-6.2402, -5.5269) (-6.2422, -5.5444) (-6.2442, -5.5619) (-6.246, -5.5794) (-6.2479, -5.597) (-6.2497, -5.6146) (-6.2514, -5.6323) (-6.2531, -5.65) (-6.2547, -5.6677) (-6.2563, -5.6855) (-6.2578, -5.7034) (-6.2593, -5.7213) (-6.2607, -5.7392) (-6.262, -5.7572) (-6.2633, -5.7752) (-6.2646, -5.7932) (-6.2656, -5.8077) (-6.2663, -5.8186) (-6.2667, -5.8259) (-6.2669, -5.8295) knots 0 0 0 0 0 0 0.00416667 0.00833333 0.0125 0.01666667 0.02083333 0.025 0.02916667 0.03333333 0.0375 0.04166667 0.04583333 0.05 0.05416667 0.05833333 0.0625 0.06666667 0.07083333 0.075 0.07916667 0.08333333 0.0875 0.09166667 0.09583333 0.1 0.10416667 0.10833333 0.1125 0.11666667 0.12083333 0.125 0.12916667 0.13333333 0.1375 0.14166667 0.14583333 0.15 0.15416667 0.15833333 0.1625 0.16666667 0.17083333 0.175 0.17916667 0.18333333 0.1875 0.19166667 0.19583333 0.2 0.20416667 0.20833333 0.2125 0.21666667 0.22083333 0.225 0.22916667 0.23333333 0.2375 0.24166667 0.24583333 0.25 0.25416667 0.25833333 0.2625 0.26666667 0.27083333 0.275 0.27916667 0.28333333 0.2875 0.29166667 0.29583333 0.3 0.30416667 0.30833333 0.3125 0.31666667 0.32083333 0.325 0.32916667 0.33333333 0.3375 0.34166667 0.34583333 0.35 0.35416667 0.35833333 0.3625 0.36666667 0.37083333 0.375 0.37916667 0.38333333 0.3875 0.39166667 0.39583333 0.4 0.40416667 0.40833333 0.4125 0.41666667 0.42083333 0.425 0.42916667 0.43333333 0.4375 0.44166667 0.44583333 0.45 0.45416667 0.45833333 0.4625 0.46666667 0.47083333 0.475 0.47916667 0.48333333 0.4875 0.49166667 0.49583333 0.5 0.50416667 0.50833333 0.5125 0.51666667 0.52083333 0.525 0.52916667 0.53333333 0.5375 0.54166667 0.54583333 0.55 0.55416667 0.55833333 0.5625 0.56666667 0.57083333 0.575 0.57916667 0.58333333 0.5875 0.59166667 0.59583333 0.6 0.60416667 0.60833333 0.6125 0.61666667 0.62083333 0.625 0.62916667 0.63333333 0.6375 0.64166667 0.64583333 0.65 0.65416667 0.65833333 0.6625 0.66666667 0.67083333 0.675 0.67916667 0.68333333 0.6875 0.69166667 0.69583333 0.7 0.70416667 0.70833333 0.7125 0.71666667 0.72083333 0.725 0.72916667 0.73333333 0.7375 0.74166667 0.74583333 0.75 0.75416667 0.75833333 0.7625 0.76666667 0.77083333 0.775 0.77916667 0.78333333 0.7875 0.79166667 0.79583333 0.8 0.80416667 0.80833333 0.8125 0.81666667 0.82083333 0.825 0.82916667 0.83333333 0.8375 0.84166667 0.84583333 0.85 0.85416667 0.85833333 0.8625 0.86666667 0.87083333 0.875 0.87916667 0.88333333 0.8875 0.89166667 0.89583333 0.9 0.90416667 0.90833333 0.9125 0.91666667 0.92083333 0.925 0.92916667 0.93333333 0.9375 0.94166667 0.94583333 0.95 0.95416667 0.95833333 0.9625 0.96666667 0.97083333 0.975 0.97916667 0.98333333 0.9875 0.99166667 0.99583333 1 1 1 1 1 1
  arc A3 (-6.2669, -5.8295) -> (-5.8295, -6.2669) centre (0, 0) ccw
  spline S3 degree 5 poles (-5.8295, -6.2669) (-5.8259, -6.2667) (-5.8186, -6.2663) (-5.8077, -6.2656) (-5.7932, -6.2646) (-5.7752, -6.2633) (-5.7572, -6.262) (-5.7392, -6.2607) (-5.7213, -6.2593) (-5.7034, -6.2578) (-5.6855, -6.2563) (-5.6677, -6.2547) (-5.65, -6.2531) (-5.6323, -6.2514) (-5.6146, -6.2497) (-5.597, -6.2479) (-5.5794, -6.246) (-5.5619, -6.2442) (-5.5444, -6.2422) (-5.5269, -6.2402) (-5.5095, -6.2382) (-5.4922, -6.2361) (-5.4749, -6.234) (-5.4576, -6.2318) (-5.4404, -6.2296) (-5.4233, -6.2273) (-5.4062, -6.225) (-5.3891, -6.2226) (-5.3721, -6.2201) (-5.3551, -6.2177) (-5.3382, -6.2151) (-5.3213, -6.2126) (-5.3045, -6.2099) (-5.2877, -6.2073) (-5.271, -6.2046) (-5.2543, -6.2018) (-5.2377, -6.199) (-5.2211, -6.1961) (-5.2046, -6.1932) (-5.1882, -6.1903) (-5.1717, -6.1873) (-5.1554, -6.1843) (-5.1391, -6.1812) (-5.1228, -6.1781) (-5.1066, -6.1749) (-5.0904, -6.1717) (-5.0743, -6.1684) (-5.0583, -6.1651) (-5.0423, -6.1618) (-5.0264, -6.1584) (-5.0105, -6.1549) (-4.9946, -6.1515) (-4.9789, -6.1479) (-4.9631, -6.1444) (-4.9475, -6.1408) (-4.9319, -6.1371) (-4.9163, -6.1334) (-4.9008, -6.1297) (-4.8854, -6.126) (-4.87, -6.1221) (-4.8547, -6.1183) (-4.8394, -6.1144) (-4.8242, -6.1105) (-4.809, -6.1065) (-4.7939, -6.1025) (-4.7789, -6.0985) (-4.7639, -6.0944) (-4.749, -6.0903) (-4.7341, -6.0861) (-4.7193, -6.0819) (-4.7046, -6.0777) (-4.6899, -6.0734) (-4.6753, -6.0691) (-4.6607, -6.0648) (-4.6462, -6.0604) (-4.6317, -6.056) (-4.6174, -6.0516) (-4.603, -6.0471) (-4.5888, -6.0426) (-4.5746, -6.038) (-4.5605, -6.0335) (-4.5464, -6.0288) (-4.5324, -6.0242) (-4.5184, -6.0195) (-4.5046, -6.0148) (-4.4908, -6.0101) (-4.477, -6.0053) (-4.4633, -6.0005) (-4.4497, -5.9957) (-4.4361, -5.9908) (-4.4226, -5.9859) (-4.4092, -5.981) (-4.3959, -5.976) (-4.3826, -5.971) (-4.3693, -5.966) (-4.3562, -5.961) (-4.3431, -5.9559) (-4.3301, -5.9509) (-4.3171, -5.9457) (-4.3042, -5.9406) (-4.2914, -5.9354) (-4.2786, -5.9302) (-4.2659, -5.925) (-4.2533, -5.9198) (-4.2408, -5.9145) (-4.2283, -5.9092) (-4.2159, -5.9039) (-4.2035, -5.8986) (-4.1913, -5.8932) (-4.1791, -5.8878) (-4.1669, -5.8824) (-4.1549, -5.877) (-4.1429, -5.8716) (-4.131, -5.8661) (-4.1191, -5.8606) (-4.1074, -5.8551) (-4.0957, -5.8496) (-4.084, -5.8441) (-4.0725, -5.8385) (-4.061, -5.833) (-4.0496, -5.8274) (-4.0383, -5.8218) (-4.027, -5.8162) (-4.0158, -5.8105) (-4.0047, -5.8049) (-3.9937, -5.7992) (-3.9827, -5.7936) (-3.9718, -5.7879) (-3.961, -5.7822) (-3.9503, -5.7765) (-3.9396, -5.7708) (-3.929, -5.765) (-3.9185, -5.7593) (-3.9081, -5.7535) (-3.8977, -5.7478) (-3.8875, -5.742) (-3.8773, -5.7363) (-3.8672, -5.7305) (-3.8571, -5.7247) (-3.8472, -5.7189) (-3.8373, -5.7131) (-3.8275, -5.7073) (-3.8177, -5.7015) (-3.8081, -5.6957) (-3.7985, -5.6899) (-3.7891, -5.6841) (-3.7796, -5.6783) (-3.7703, -5.6725) (-3.7611, -5.6666) (-3.7519, -5.6608) (-3.7428, -5.655) (-3.7338, -5.6492) (-3.7249, -5.6434) (-3.7161, -5.6376) (-3.7073, -5.6318) (-3.6987, -5.626) (-3.6901, -5.6203) (-3.6816, -5.6145) (-3.6732, -5.6087) (-3.6648, -5.603) (-3.6566, -5.5972) (-3.6484, -5.5915) (-3.6404, -5.5857) (-3.6324, -5.58) (-3.6244, -5.5743) (-3.6166, -5.5686) (-3.6089, -5.5629) (-3.6012, -5.5573) (-3.5937, -5.5516) (-3.5862, -5.546) (-3.5788, -5.5404) (-3.5715, -5.5348) (-3.5643, -5.5292) (-3.5571, -5.5236) (-3.5501, -5.5181) (-3.5431, -5.5126) (-3.5363, -5.5071) (-3.5295, -5.5016) (-3.5228, -5.4962) (-3.5162, -5.4908) (-3.5097, -5.4854) (-3.5033, -5.48) (-3.497, -5.4747) (-3.4907, -5.4694) (-3.4846, -5.4641) (-3.4785, -5.4589) (-3.4725, -5.4537) (-3.4667, -5.4485) (-3.4609, -5.4434) (-3.4552, -5.4383) (-3.4496, -5.4332) (-3.4441, -5.4282) (-3.4387, -5.4232) (-3.4333, -5.4183) (-3.4281, -5.4134) (-3.423, -5.4085) (-3.4179, -5.4037) (-3.413, -5.399) (-3.4081, -5.3943) (-3.4034, -5.3896) (-3.3987, -5.385) (-3.3941, -5.3804) (-3.3897, -5.3759) (-3.3853, -5.3715) (-3.381, -5.3671) (-3.3768, -5.3628) (-3.3727, -5.3585) (-3.3687, -5.3543) (-3.3648, -5.3501) (-3.361, -5.3461) (-3.3573, -5.342) (-3.3537, -5.3381) (-3.3502, -5.3342) (-3.3468, -5.3304) (-3.3435, -5.3267) (-3.3403, -5.323) (-3.3372, -5.3195) (-3.3342, -5.316) (-3.3313, -5.3126) (-3.3285, -5.3092) (-3.3258, -5.306) (-3.3231, -5.3029) (-3.3206, -5.2998) (-3.3182, -5.2968) (-3.3159, -5.294) (-3.3137, -5.2912) (-3.3116, -5.2885) (-3.3096, -5.2859) (-3.3077, -5.2835) (-3.3059, -5.2811) (-3.3042, -5.2789) (-3.3026, -5.2767) (-3.3012, -5.2747) (-3.2998, -5.2728) (-3.2985, -5.2711) (-3.2973, -5.2694) (-3.2963, -5.2679) (-3.2953, -5.2665) (-3.2945, -5.2653) (-3.2937, -5.2642) (-3.2931, -5.2633) (-3.2927, -5.2626) (-3.2924, -5.2622) (-3.2922, -5.262) (-3.2921, -5.2619) knots -1 -1 -1 -1 -1 -1 -0.99583333 -0.99166667 -0.9875 -0.98333333 -0.97916667 -0.975 -0.97083333 -0.96666667 -0.9625 -0.95833333 -0.95416667 -0.95 -0.94583333 -0.94166667 -0.9375 -0.93333333 -0.92916667 -0.925 -0.92083333 -0.91666667 -0.9125 -0.90833333 -0.90416667 -0.9 -0.89583333 -0.89166667 -0.8875 -0.88333333 -0.87916667 -0.875 -0.87083333 -0.86666667 -0.8625 -0.85833333 -0.85416667 -0.85 -0.84583333 -0.84166667 -0.8375 -0.83333333 -0.82916667 -0.825 -0.82083333 -0.81666667 -0.8125 -0.80833333 -0.80416667 -0.8 -0.79583333 -0.79166667 -0.7875 -0.78333333 -0.77916667 -0.775 -0.77083333 -0.76666667 -0.7625 -0.75833333 -0.75416667 -0.75 -0.74583333 -0.74166667 -0.7375 -0.73333333 -0.72916667 -0.725 -0.72083333 -0.71666667 -0.7125 -0.70833333 -0.70416667 -0.7 -0.69583333 -0.69166667 -0.6875 -0.68333333 -0.67916667 -0.675 -0.67083333 -0.66666667 -0.6625 -0.65833333 -0.65416667 -0.65 -0.64583333 -0.64166667 -0.6375 -0.63333333 -0.62916667 -0.625 -0.62083333 -0.61666667 -0.6125 -0.60833333 -0.60416667 -0.6 -0.59583333 -0.59166667 -0.5875 -0.58333333 -0.57916667 -0.575 -0.57083333 -0.56666667 -0.5625 -0.55833333 -0.55416667 -0.55 -0.54583333 -0.54166667 -0.5375 -0.53333333 -0.52916667 -0.525 -0.52083333 -0.51666667 -0.5125 -0.50833333 -0.50416667 -0.5 -0.49583333 -0.49166667 -0.4875 -0.48333333 -0.47916667 -0.475 -0.47083333 -0.46666667 -0.4625 -0.45833333 -0.45416667 -0.45 -0.44583333 -0.44166667 -0.4375 -0.43333333 -0.42916667 -0.425 -0.42083333 -0.41666667 -0.4125 -0.40833333 -0.40416667 -0.4 -0.39583333 -0.39166667 -0.3875 -0.38333333 -0.37916667 -0.375 -0.37083333 -0.36666667 -0.3625 -0.35833333 -0.35416667 -0.35 -0.34583333 -0.34166667 -0.3375 -0.33333333 -0.32916667 -0.325 -0.32083333 -0.31666667 -0.3125 -0.30833333 -0.30416667 -0.3 -0.29583333 -0.29166667 -0.2875 -0.28333333 -0.27916667 -0.275 -0.27083333 -0.26666667 -0.2625 -0.25833333 -0.25416667 -0.25 -0.24583333 -0.24166667 -0.2375 -0.23333333 -0.22916667 -0.225 -0.22083333 -0.21666667 -0.2125 -0.20833333 -0.20416667 -0.2 -0.19583333 -0.19166667 -0.1875 -0.18333333 -0.17916667 -0.175 -0.17083333 -0.16666667 -0.1625 -0.15833333 -0.15416667 -0.15 -0.14583333 -0.14166667 -0.1375 -0.13333333 -0.12916667 -0.125 -0.12083333 -0.11666667 -0.1125 -0.10833333 -0.10416667 -0.1 -0.09583333 -0.09166667 -0.0875 -0.08333333 -0.07916667 -0.075 -0.07083333 -0.06666667 -0.0625 -0.05833333 -0.05416667 -0.05 -0.04583333 -0.04166667 -0.0375 -0.03333333 -0.02916667 -0.025 -0.02083333 -0.01666667 -0.0125 -0.00833333 -0.00416667 0 0 0 0 0 0
  line L6 (-3.2921, -5.2619) -> (-3.2915, -5.2609)
  line L7 (-3.2915, -5.2609) -> (-2.4969, -3.9908)
  arc A4 (-2.4969, -3.9908) -> (-1.0563, -4.5874) centre (0, 0) ccw
  line L8 (-1.0563, -4.5874) -> (-1.3925, -6.0475)
  line L9 (-1.3925, -6.0475) -> (-1.3928, -6.0486)